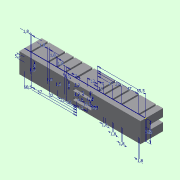
# Autodesk Inventor part: Distance_test_rig
Saved by Autodesk Inventor 2015 (Build 190159000, 159)
## iProperties
Created: 2015-05-18
Part Number: Distance_test_rig
Material: Generic
Document SubType Name: Modeling
Designer: Openlab
Density: 1 g/cm^3
Appearance: Default
Author: Openlab
Autodesk Inventor part; units mm, degrees
ref_plane "YZ Plane" through (0, 0, 0) normal (1, 0, 0) x (0, 1, 0)
ref_plane "XZ Plane" through (0, 0, 0) normal (0, 1, 0) x (-1, 0, 0)
ref_plane "XY Plane" through (0, 0, 0) normal (0, 0, 1) x (1, 0, 0)
sketch "Sketch1" plane through (0, 0, 0) normal (0, 1, 0) x (-1, 0, 0)
  line L0 (73.75, -5.25) -> (61.25, -5.25)
  line L1 (61.25, -5.25) -> (61.25, -17.75)
  line L2 (61.25, -17.75) -> (73.75, -17.75)
  line L3 (73.75, -17.75) -> (73.75, -5.25)
  line L4 (140, 0) -> (0, 0)
  line L5 (0, 0) -> (0, -23)
  line L6 (0, -23) -> (140, -23)
  line L7 (140, -23) -> (140, 0)
  line L8 (77.3838, -11.5) -> (49.3838, -11.5) construction
  line L9 (67.5, -2.25) -> (67.5, -23.25) construction
  line L10 (91.5, 0) -> (91.5, -23)
  line L11 (93.3, -23) -> (93.3, 0)
  line L12 (101.5, 0) -> (101.5, -23)
  line L13 (103.3, -23) -> (103.3, 0)
  line L14 (111.5, 0) -> (111.5, -23)
  line L15 (113.3, 0) -> (113.3, -23)
  line L16 (131.5, 0) -> (131.5, -23)
  line L17 (133.3, -23) -> (133.3, 0)
  line L18 (81.5, -8.9) -> (140, -8.9)
  line L19 (140, -14.1) -> (81.5, -14.1)
  line L20 (48.5, -23) -> (48.5, 0)
  line L21 (46.7, 0) -> (46.7, -23)
  line L22 (38.5, 0) -> (38.5, -23)
  line L23 (36.7, 0) -> (36.7, -23)
  line L24 (28.5, 0) -> (28.5, -23)
  line L25 (26.7, 0) -> (26.7, -23)
  line L26 (8.5, 0) -> (8.5, -23)
  line L27 (6.7, -23) -> (6.7, 0)
  line L28 (53.5, -8.9) -> (0, -8.9)
  line L29 (53.5, -14.1) -> (0, -14.1)
  line L30 (91.5, -15.5) -> (90, -15.5)
  line L31 (90, -15.5) -> (90, -7.5)
  line L32 (90, -7.5) -> (91.5, -7.5)
  line L33 (101.5, -15.5) -> (100, -15.5)
  line L34 (100, -15.5) -> (100, -7.5)
  line L35 (100, -7.5) -> (101.5, -7.5)
  line L36 (111.5, -15.5) -> (110, -15.5)
  line L37 (110, -15.5) -> (110, -7.5)
  line L38 (110, -7.5) -> (111.5, -7.5)
  line L39 (131.5, -15.5) -> (130, -15.5)
  line L40 (130, -15.5) -> (130, -7.5)
  line L41 (130, -7.5) -> (131.5, -7.5)
  line L42 (79.5, 0) -> (79.5, -23)
  line L43 (81.5, -23) -> (81.5, 0)
  line L44 (55.5, 0) -> (55.5, -23)
  line L45 (53.5, -23) -> (53.5, 0)
  line L46 (79.5, -13) -> (73.75, -13)
  line L47 (73.75, -10) -> (79.5, -10)
  line L48 (61.25, -13) -> (55.5, -13)
  line L49 (55.5, -10) -> (61.25, -10)
  line L50 (73.75, -17.75) -> (77.95, -17.75)
  line L51 (77.95, -17.75) -> (77.95, -14.55)
  line L52 (77.95, -14.55) -> (73.75, -14.55)
  line L53 (73.75, -14.55) -> (61.25, -14.55)
  line L54 (56.65, -14.55) -> (56.65, -17.75)
  line L55 (56.65, -17.75) -> (59.85, -17.75)
  line L56 (59.85, -14.55) -> (56.65, -14.55)
  line L57 (59.85, -5.25) -> (56.65, -5.25)
  line L58 (56.65, -5.25) -> (56.65, -8.45)
  line L59 (56.65, -8.45) -> (59.85, -8.45)
  line L60 (61.25, -8.45) -> (73.75, -8.45)
  line L61 (77.95, -8.45) -> (77.95, -5.25)
  line L62 (73.75, -5.25) -> (77.95, -5.25)
  line L63 (77.95, -8.45) -> (73.75, -8.45)
  line L64 (59.85, -17.75) -> (59.85, -14.55)
  line L65 (59.85, -8.45) -> (59.85, -5.25)
  line L66 (61.25, -17.75) -> (59.85, -17.75)
  line L67 (61.25, -14.55) -> (59.85, -14.55)
  line L68 (61.25, -8.45) -> (59.85, -8.45)
  line L69 (61.25, -5.25) -> (59.85, -5.25)
  point P0 (133.3, -8.9)
  point P1 (133.3, -14.1)
  point P2 (131.5, -8.9)
  point P3 (131.5, -14.1)
  point P4 (113.3, -8.9)
  point P5 (111.5, -8.9)
  point P6 (113.3, -14.1)
  point P7 (111.5, -14.1)
  point P8 (103.3, -8.9)
  point P9 (101.5, -8.9)
  point P10 (103.3, -14.1)
  point P11 (101.5, -14.1)
  point P12 (93.3, -8.9)
  point P13 (91.5, -8.9)
  point P14 (93.3, -14.1)
  point P15 (91.5, -14.1)
  point P16 (48.5, -8.9)
  point P17 (46.7, -8.9)
  point P18 (48.5, -14.1)
  point P19 (46.7, -14.1)
  point P20 (38.5, -14.1)
  point P21 (36.7, -14.1)
  point P22 (36.7, -8.9)
  point P23 (38.5, -8.9)
  point P24 (28.5, -8.9)
  point P25 (26.7, -8.9)
  point P26 (26.7, -14.1)
  point P27 (28.5, -14.1)
  point P28 (8.5, -14.1)
  point P29 (6.7, -14.1)
  point P30 (6.7, -8.9)
  point P31 (8.5, -8.9)
  point P32 (67.5, -11.5)
  point P33 (90, -14.1)
  point P34 (90, -8.9)
  point P35 (130, -14.1)
  point P36 (130, -8.9)
  point P37 (110, -14.1)
  point P38 (110, -8.9)
  point P39 (100, -8.9)
  point P40 (100, -14.1)
  dimension "d12" = 5.2
  dimension "d25" = 5.2
  dimension "d0" = 12.5
  dimension "d1" = 12.5
  dimension "d3" = 23
  dimension "d5" = 1.8
  dimension "d7" = 1.8
  dimension "d9" = 1.8
  dimension "d11" = 1.8
  dimension "d18" = 1.8
  dimension "d20" = 1.8
  dimension "d22" = 1.8
  dimension "d24" = 1.8
  dimension "d32" = 1.5
  dimension "d33" = 8
  dimension "d36" = 8
  dimension "d37" = 1.5
  dimension "d38" = 1.5
  dimension "d39" = 1.5
  dimension "d43" = 2
  dimension "d45" = 2
  dimension "d52" = 12
  dimension "d57" = 12
  dimension "d62" = 3
  dimension "d63" = 3
  dimension "d66" = 12
  dimension "d67" = 22
  dimension "d68" = 32
  dimension "d69" = 52
  dimension "d70" = 60.5
  dimension "d71" = 7
  dimension "d72" = 17
  dimension "d73" = 27
  dimension "d74" = 47
  dimension "d75" = 55.5
  dimension "d76" = 4.2
  dimension "d77" = 3.2
  dimension "d78" = 3.2
  dimension "d79" = 1.4
  dimension "d80" = 3.2
  constraints: 128 end point, 90 point on line, 27 vertical, 15 perpendicular, 10 horizontal, 9 parallel, 1 coincident, 104 other
  measures "d0" distance of L2.end L1.end
  measures "d1" distance of L0.end L1.end
  measures "d3" distance of L5.end L5.start
  measures "d5" distance between parallel lines of L10 L11
  measures "d7" distance between parallel lines of L13 L12
  measures "d9" distance between parallel lines of L14 L15
  measures "d11" distance between parallel lines of L16 L17
  measures "d18" distance between parallel lines of L21 L20
  measures "d20" distance between parallel lines of L23 L22
  measures "d22" distance between parallel lines of L25 L24
  measures "d24" distance between parallel lines of L27 L26
  measures "d32" distance of L31.end L32.end
  measures "d33" distance of L30.end L31.end
  measures "d36" distance of L39.end L40.end
  measures "d37" distance of L39.start L39.end
  measures "d38" distance of L36.start L36.end
  measures "d39" distance of L33.start L33.end
  measures "d43" distance between parallel lines of L43 L42
  measures "d45" distance between parallel lines of L45 L44
  measures "d52" distance between parallel lines of L44 L9
  measures "d57" distance between parallel lines of L42 L9
  measures "d62" distance between parallel lines of L47 L46
  measures "d63" distance between parallel lines of L49 L48
  measures "d66" distance between parallel lines of L10 L42
  measures "d67" distance between parallel lines of L12 L42
  measures "d68" distance between parallel lines of L14 L42
  measures "d69" distance between parallel lines of L16 L42
  measures "d70" distance between parallel lines of L7 L42
  measures "d71" distance between parallel lines of L20 L44
  measures "d72" distance between parallel lines of L22 L44
  measures "d73" distance between parallel lines of L24 L44
  measures "d74" distance between parallel lines of L26 L44
  measures "d75" distance between parallel lines of L5 L44
  measures "d76" distance of L2.end L50.end
  measures "d77" distance of L50.end L51.end
  measures "d78" distance of L61.start L61.end
  measures "d79" distance between parallel lines of L64 L1
  measures "d80" distance of L54.end L55.end
extrude "Extrusion10" add sketch "Sketch1" against normal blind 6 contours L0 L69 L57 L58 L59 L68 L1 L49 L44 L4 L42 L47 L3 L63 L61 L62 | L3 L53 L1 L60 | L47 L42 L46 L3 | L1 L48 L44 L49 | L46 L42 L6 L44 L48 L1 L67 L56 L54 L55 L66 L2 L50 L51 L52 L3 | L42 L4 L43 L6 | L44 L6 L45 L4 | L4 L10 L32 L31 L18 L43 | L45 L28 L20 L4 | L43 L19 L31 L30 L10 L6 | L4 L11 L18 L10 | L18 L31 L19 L43 | L6 L20 L29 L45 | L20 L28 L21 L4 | L45 L29 L20 L28 | L10 L19 L11 L6 | L4 L12 L35 L34 L18 L11 | L10 L18 L31 L32 | L18 L10 L19 L31 | L6 L21 L29 L20 | L21 L28 L22 L4 | L20 L29 L21 L28 | L11 L19 L34 L33 L12 L6 | L30 L31 L19 L10 | L4 L13 L18 L12 | L18 L34 L19 L11 | L11 L19 L10 L18 | L6 L22 L29 L21 | L22 L28 L23 L4 | L21 L29 L22 L28 | L12 L19 L13 L6 | L4 L14 L38 L37 L18 L13 | L12 L18 L34 L35 | L18 L12 L19 L34 | L6 L23 L29 L22 | L23 L28 L24 L4 | L22 L29 L23 L28 | L13 L19 L37 L36 L14 L6 | L33 L34 L19 L12 | L4 L15 L18 L14 | L18 L37 L19 L13 | L13 L19 L12 L18 | L6 L24 L29 L23 | L24 L28 L25 L4 | L23 L29 L24 L28 | L14 L19 L15 L6 | L4 L16 L41 L40 L18 L15 | L14 L18 L37 L38 | L18 L14 L19 L37 | L6 L25 L29 L24 | L25 L28 L26 L4 | L24 L29 L25 L28 | L15 L19 L40 L39 L16 L6 | L36 L37 L19 L14 | L4 L17 L18 L16 | L18 L40 L19 L15 | L15 L19 L14 L18 | L6 L26 L29 L25 | L26 L28 L27 L4 | L25 L29 L26 L28 | L16 L19 L17 L6 | L4 L7 L18 L17 | L16 L18 L40 L41 | L18 L16 L19 L40 | L6 L27 L29 L26 | L27 L28 L5 L4 | L26 L29 L27 L28 | L17 L19 L7 L6 | L39 L40 L19 L16 | L18 L7 L19 L17 | L17 L19 L16 L18 | L6 L5 L29 L27 | L27 L29 L5 L28
extrude "Extrusion11" add sketch "Sketch1" against normal blind 3 contours L3 L60 L1 L0 | L1 L68 L65 L69 | L3 L2 L1 L53 | L1 L66 L64 L67
extrude "Extrusion12" add sketch "Sketch1" along normal blind 5 contours L0 L69 L57 L58 L59 L68 L1 L49 L44 L4 L42 L47 L3 L63 L61 L62 | L1 L68 L65 L69 | L47 L42 L46 L3 | L1 L48 L44 L49 | L46 L42 L6 L44 L48 L1 L67 L56 L54 L55 L66 L2 L50 L51 L52 L3 | L1 L66 L64 L67 | L4 L10 L32 L31 L18 L43 | L45 L28 L20 L4 | L43 L19 L31 L30 L10 L6 | L18 L31 L19 L43 | L6 L20 L29 L45 | L45 L29 L20 L28 | L4 L12 L35 L34 L18 L11 | L21 L28 L22 L4 | L11 L19 L34 L33 L12 L6 | L18 L34 L19 L11 | L6 L22 L29 L21 | L21 L29 L22 L28 | L4 L14 L38 L37 L18 L13 | L23 L28 L24 L4 | L13 L19 L37 L36 L14 L6 | L18 L37 L19 L13 | L6 L24 L29 L23 | L23 L29 L24 L28 | L4 L16 L41 L40 L18 L15 | L25 L28 L26 L4 | L15 L19 L40 L39 L16 L6 | L18 L40 L19 L15 | L6 L26 L29 L25 | L25 L29 L26 L28 | L4 L7 L18 L17 | L27 L28 L5 L4 | L17 L19 L7 L6 | L18 L7 L19 L17 | L6 L5 L29 L27 | L27 L29 L5 L28
extrude "Extrusion13" add sketch "Sketch1" along normal blind 20 contours L0 L69 L57 L58 L59 L68 L1 L49 L44 L4 L42 L47 L3 L63 L61 L62 | L1 L68 L65 L69 | L46 L42 L6 L44 L48 L1 L67 L56 L54 L55 L66 L2 L50 L51 L52 L3 | L1 L66 L64 L67 | L4 L10 L32 L31 L18 L43 | L45 L28 L20 L4 | L43 L19 L31 L30 L10 L6 | L6 L20 L29 L45 | L4 L12 L35 L34 L18 L11 | L21 L28 L22 L4 | L11 L19 L34 L33 L12 L6 | L6 L22 L29 L21 | L4 L14 L38 L37 L18 L13 | L23 L28 L24 L4 | L13 L19 L37 L36 L14 L6 | L6 L24 L29 L23 | L4 L16 L41 L40 L18 L15 | L25 L28 L26 L4 | L15 L19 L40 L39 L16 L6 | L6 L26 L29 L25 | L4 L7 L18 L17 | L27 L28 L5 L4 | L17 L19 L7 L6 | L6 L5 L29 L27
extrude "Extrusion14" add sketch "Sketch1" along normal blind 2.5 contours L3 L60 L1 L0 | L3 L53 L1 L60 | L3 L2 L1 L53
body "Solid3"
